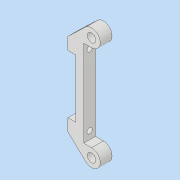
# Autodesk Inventor part: relayHolder2
Saved by Autodesk Inventor 2017 (Build 210142000, 142)
## iProperties
Created: 2019-07-11
Part Number: relayHolder2
Material: ABS Plastic
Document SubType Name: Modeling
Designer: techn
Density: 1.06 g/cm^3
Appearance: Smooth - White
Author: techn
Autodesk Inventor part; units mm, degrees
ref_plane "YZ Plane" through (0, 0, 0) normal (1, 0, 0) x (0, 1, 0)
ref_plane "XZ Plane" through (0, 0, 0) normal (0, 1, 0) x (-1, 0, 0)
ref_plane "XY Plane" through (0, 0, 0) normal (0, 0, 1) x (1, 0, 0)
sketch "Sketch1" plane through (0, 0, 0) normal (0, 0, 1) x (1, 0, 0)
  circle A0 centre (0, 0) radius 1.7145
  circle A1 centre (0, 41.91) radius 1.7145
  arc A2 (0, 38.4175) -> (-2.4156, 44.4323) centre (0, 41.91) ccw
  arc A3 (-2.4156, -2.5223) -> (0, 3.4925) centre (0, 0) ccw
  line L0 (0, 3.4925) -> (-3.175, 3.4925)
  line L1 (-3.175, 3.4925) -> (-3.175, 38.4175)
  line L2 (-3.175, 38.4175) -> (0, 38.4175)
  line L3 (-9.525, 37.6238) -> (-9.525, 4.2862)
  line L4 (-9.525, 4.2862) -> (-2.4156, -2.5223)
  line L5 (-9.525, 37.6238) -> (-2.4156, 44.4323)
  dimension "d0" = 3.429
  dimension "d1" = 3.429
  dimension "d2" = 6.985
  dimension "d3" = 6.985
  dimension "d4" = 3.175
  dimension "d5" = 41.91
  dimension "d6" = 33.3375
  dimension "d13" = 9.525
  constraints: 12 end point, 4 centre point, 4 point on circle, 3 coincident, 3 tangent, 1 equal length, 1 horizontal, 1 perpendicular, 1 vertical, 1 vertical alignment
  measures "d0" diameter of A0
  measures "d1" diameter of A1
  measures "d2" diameter of A2
  measures "d3" diameter of A3
  measures "d4" distance of L0.start L0.end
  measures "d5" distance of point (0, 0) A1.centre
  measures "d6" distance of L3.start L3.end
  measures "d13" horizontal distance of point (0, 0) L3.end
extrude "Extrusion1" add sketch "Sketch1" along normal blind 4.7625
sketch "Sketch2" plane through (-9.525, 4.2862, 0) normal (-1, 0, 0) x (0, 0, 1)
  circle A0 centre (2.3812, 30.9563) radius 1.0795
  circle A1 centre (2.3812, 2.3813) radius 1.0795
  line L0 (0, 33.3375) -> (4.7625, 33.3375) construction
  line L1 (2.3812, 30.9563) -> (2.3812, 2.3813) construction
  line L2 (0, 0) -> (0, 33.3375) construction
  point P0 (0, -4.2862)
  point P1 (2.3813, 33.3375)
  point P2 (2.3813, 16.6688)
  point P3 (0, 16.6688)
  dimension "d9" = 28.575
  dimension "d10" = 2.159
  constraints: 3 midpoint, 2 centre point, 2 end point, 2 vertical alignment, 1 equal radius, 1 horizontal alignment, 1 vertical
  measures "d9" distance of L1.end L1.start
  measures "d10" diameter of A0
extrude "Extrusion2" cut sketch "Sketch2" against normal through all
sketch "Sketch3" plane through (-9.525, 4.2862, 0) normal (-1, 0, 0) x (0, 0, 1)
  circle A0 centre (2.3812, 30.9563) radius 1.0795 construction
  circle A1 centre (2.3812, 2.3813) radius 1.0795 construction
  line L0 (0, 0) -> (0, 33.3375) construction
  line L1 (0, 0) -> (4.7625, 0) construction
  line L2 (4.7625, 33.3375) -> (4.7625, 0) construction
  line L3 (0, 33.3375) -> (4.7625, 33.3375) construction
  line L4 (4.7625, -0.7937) -> (4.7625, 34.1313) projected
  line L5 (0, 28.4163) -> (4.7625, 28.4163)
  line L6 (4.7625, 28.4163) -> (4.7625, 4.9212)
  line L7 (4.7625, 4.9212) -> (0, 4.9212)
  line L8 (0, 4.9212) -> (0, 28.4163)
  point P0 (0, -4.2862)
  point P1 (4.7625, 16.6688)
  point P2 (4.7625, 16.6688)
  dimension "d14" = 23.495
  constraints: 8 end point, 2 midpoint, 2 parallel, 2 point on line, 1 coincident, 1 horizontal, 1 perpendicular
  measures "d14" distance between parallel lines of L7 L5
extrude "Extrusion3" cut sketch "Sketch3" against normal blind 3.175
body "Solid1"
